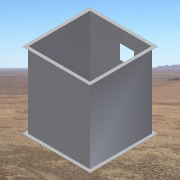
# Autodesk Inventor part: housing
Saved by Autodesk Inventor 2014 SP1 (Build 180222100, 222)
## iProperties
Created: 2014-03-11
Part Number: housing
Material: Aluminum 6061
Document SubType Name: Modeling
Designer: Dave
Density: 2.71 g/cm^3
Appearance: Aluminum - Flat
Mass: 15486.1 g
Surface Area: 45813.7 cm^2
Volume: 5714.43 cm^3
Author: Dave
Autodesk Inventor part; units mm, degrees
ref_plane "YZ Plane" through (0, 0, 0) normal (1, 0, 0) x (0, 1, 0)
ref_plane "XZ Plane" through (0, 0, 0) normal (0, 1, 0) x (-1, 0, 0)
ref_plane "XY Plane" through (0, 0, 0) normal (0, 0, 1) x (1, 0, 0)
sketch "Sketch1" plane through (0, 0, 0) normal (0, 1, 0) x (-1, 0, 0)
  line L0 (0, 0) -> (850, 0)
  line L1 (850, 0) -> (850, 850)
  line L2 (850, 850) -> (0, 850)
  line L3 (0, 850) -> (0, 0)
  dimension "d0" = 850
  dimension "d1" = 850
  constraints: 8 end point, 2 parallel, 1 horizontal, 1 perpendicular
  measures "d0" distance of L0.start L0.end
  measures "d1" distance of L2.end L0.start
extrude "Extrusion1" add sketch "Sketch1" along normal blind 950
sketch "Sketch2" plane through (0, 950, 0) normal (0, 1, 0) x (1, 0, 0)
  line L0 (0, 0) -> (-850, 0) projected
  line L1 (-850, 0) -> (-850, -850) projected
  line L2 (-850, -850) -> (0, -850) projected
  line L3 (0, -850) -> (0, 0) projected
  line L4 (-810, -40) -> (-40, -40)
  line L5 (-40, -40) -> (-40, -810)
  line L6 (-40, -810) -> (-810, -810)
  line L7 (-810, -810) -> (-810, -40)
  dimension "d4" = 40
  constraints: 8 end point, 3 other
  measures "d4" distance between parallel lines of L4 L0
extrude "Extrusion2" cut sketch "Sketch2" against normal blind 1000 contours L4 L5 L6 L7
sketch "Sketch3" plane through (-850, 0, 850) normal (0, 0, 1) x (1, 0, 0)
  line L0 (0, 0) -> (850, 0) projected
  line L1 (850, 0) -> (850, 950) projected
  line L2 (0, 950) -> (850, 950) projected
  line L3 (0, 0) -> (0, 950) projected
  line L4 (0, 2.54) -> (850, 2.54)
  line L5 (850, 2.54) -> (850, 947.46)
  line L6 (850, 947.46) -> (0, 947.46)
  line L7 (0, 947.46) -> (0, 2.54)
  dimension "d7" = 2.54
  dimension "d8" = 2.54
  constraints: 8 end point, 2 parallel, 2 point on line, 1 horizontal, 1 perpendicular
  measures "d7" distance between parallel lines of L6 L2
  measures "d8" distance between parallel lines of L0 L4
extrude "Extrusion3" cut sketch "Sketch3" against normal blind 37.5 contours L3 L6 L1 L4
sketch "Sketch4" plane through (0, 0, 0) normal (0, 0, -1) x (-1, 0, 0)
  line L0 (0, 0) -> (850, 0) projected
  line L1 (850, 0) -> (850, 950) projected
  line L2 (0, 950) -> (850, 950) projected
  line L3 (0, 0) -> (0, 950) projected
  line L4 (0, 2.54) -> (850, 2.54)
  line L5 (850, 2.54) -> (850, 947.46)
  line L6 (850, 947.46) -> (0, 947.46)
  line L7 (0, 947.46) -> (0, 2.54)
  dimension "d11" = 2.54
  dimension "d12" = 2.54
  constraints: 8 end point, 2 parallel, 2 point on line, 1 horizontal, 1 perpendicular
  measures "d11" distance between parallel lines of L6 L2
  measures "d12" distance between parallel lines of L0 L4
extrude "Extrusion4" cut sketch "Sketch4" against normal blind 37.5 contours L3 L6 L1 L4
sketch "Sketch5" plane through (0, 0, 37.5) normal (0, 0, -1) x (-1, 0, 0)
  line L0 (850, 2.54) -> (0, 2.54) projected
  line L1 (0, 947.46) -> (37.5, 947.46)
  line L2 (37.5, 947.46) -> (37.5, 2.54)
  line L3 (37.5, 2.54) -> (0, 2.54)
  line L4 (0, 2.54) -> (0, 947.46)
  line L5 (850, 947.46) -> (812.5, 947.46)
  line L6 (812.5, 947.46) -> (812.5, 2.54)
  line L7 (812.5, 2.54) -> (850, 2.54)
  line L8 (850, 2.54) -> (850, 947.46)
  point P0 (0, 0)
  dimension "d15" = 37.5
  dimension "d16" = 37.5
  constraints: 16 end point, 4 parallel, 2 horizontal, 2 perpendicular, 2 point on line
  measures "d15" distance between parallel lines of L2 L4
  measures "d16" distance between parallel lines of L6 L8
extrude "Extrusion5" cut sketch "Sketch5" against normal blind 1000
sketch "Sketch6" plane through (0, 950, 0) normal (0, 1, 0) x (1, 0, 0)
  line L0 (0, 0) -> (-850, 0) projected
  line L1 (-850, 0) -> (-850, -850) projected
  circle A0 centre (-835, -15) radius 5.0825
  point P0 (-165, -15)
  point P1 (-835, -685)
  point P2 (-165, -685)
  dimension "d19" = 15
  dimension "d20" = 15
  dimension "d23" = 670
  dimension "d26" = 670
  constraints: 1 centre point, 1 horizontal, 1 vertical, 3 other
  measures "d19" distance from line of A0.centre L0
  measures "d20" distance from line of A0.centre L1
  measures "d23" distance of A0.centre point (-165, -15)
  measures "d26" distance of A0.centre point (-835, -685)
hole "Hole1" at (-835, 950, 685) at (-835, 950, 15) at (-165, 950, 15) at (-165, 950, 685) direction (0, -1, 0) diameter 6.35 end through all
sketch "Sketch7" plane through (0, 0, 37.5) normal (0, 0, -1) x (-1, 0, 0)
  line L0 (37.5, 947.46) -> (37.5, 2.54) projected
  line L1 (257.5, 604.8881) -> (437.5, 604.8881)
  line L2 (437.5, 604.8881) -> (437.5, 784.8881)
  line L3 (437.5, 784.8881) -> (257.5, 784.8881)
  line L4 (257.5, 784.8881) -> (257.5, 604.8881)
  point P0 (0, 0)
  dimension "d36" = 220
  dimension "d37" = 180
  dimension "d38" = 180
  constraints: 8 end point, 2 parallel, 1 horizontal, 1 perpendicular
  measures "d36" distance between parallel lines of L4 L0
  measures "d37" distance of L3.end L1.start
  measures "d38" distance of L2.end L3.end
extrude "Extrusion6" cut sketch "Sketch7" against normal blind 10
body "Solid1"
